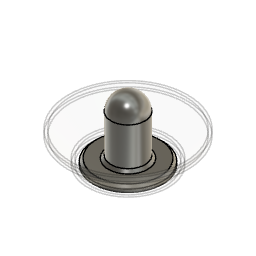
Moka Pot Coffee Funnel and Tamper (Autodesk Fusion 360 design; units mm, degrees)
Autodesk Fusion 360 part; units mm, degrees
sketch "Sketch1" plane through (0, 0, 0) normal (0, 1, 0) x (1, 0, 0)
  line L0 (0, 0) -> (-29.75, 0) construction
  line L1 (-29.75, 0) -> (-29.75, -4)
  line L2 (-29.75, -4) -> (-44, -18.5242)
  line L3 (-44, -18.5242) -> (-42, -18.5242)
  line L4 (-42, -18.5242) -> (-27.75, -4)
  line L5 (-27.75, -4) -> (-27.75, 0)
  line L6 (-29.75, 0) -> (-27.75, 0)
  line L7 (-44, -18.5242) -> (-44, -22.5242)
  line L8 (-44, -22.5242) -> (-42, -22.5242)
  line L9 (-42, -22.5242) -> (-42, -18.5242)
  dimension "d2" = 4
  dimension "d3" = 29.75
  dimension "d4" = 42
  dimension "d5" = 14.5242
  dimension "d7" = 4
  dimension "d8" = 2
  constraint coincident L0.start origin
  constraint horizontal L0
  constraint perpendicular L0 L1
  constraint parallel L0 L3
  constraint parallel L2 L4
  constraint coincident L0 L5.end
  constraint perpendicular L0 L5
  constraint equal L3 L6
  constraint perpendicular L3 L7
  constraint perpendicular L7 L8
  constraint perpendicular L3 L9
  measures "d2" distance of L4.end L5.end
  measures "d3" distance of L0.start L0.end
  measures "d4" horizontal distance of L0.start L3.end
  measures "d5" vertical distance of L1.end L2.end
  measures "d7" distance of L2.end L7.end
  measures "d8" distance of L7.end L8.end
revolve "Revolve1" add sketch "Sketch1" angle 360 about axis through (0, 0, 1.75) along (0, 0, 1) makes body 1
cylinder "CylinderPrimitive1" add diameter 51 height 4 placed x (1, 0, 0) y (0, 1, 0) z (0, 0, 1) at (0, 0, 0) separate body makes body 2 in component "Tamper"
cylinder "CylinderPrimitive2" add diameter 25 height 30 placed x (1, 0, 0) y (0, 1, 0) z (0, 0, 1) at (0, 0, 4) bodies 2 in component "Tamper"
sphere "SpherePrimitive1" add diameter 25 placed x (-1, 0, 0) y (0, -1, 0) z (0, 0, 1) at (0, 0, 34) bodies 2 in component "Tamper"
chamfer "Chamfer1" distance 2 angle 45 1 edges at (-23.7743, -9.2212, 4) on bodies 2 in component "Tamper"
chamfer "Chamfer1" distance 2 angle 45 1 edges at (-11.6541, 4.5202, 4) on bodies 2 in component "Tamper"
component "Tamper" placed x (1, 0, 0) y (0, 1, 0) z (0, 0, 1) at (0, 0, 0)
equation "d3 = ( 59.5 / 2 ) * 1 mm"
equation "d4 = ( 84 / 2 ) * 1 mm"
named bodies: "Moka Pot Coffee Funnel", "Tamper"
